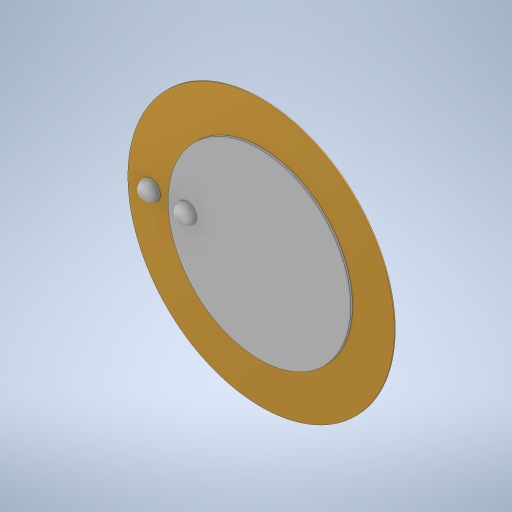
# Autodesk Inventor part: Piezo
Saved by Autodesk Inventor 2023 (Build 270158000, 158)
## iProperties
Created: 2023-02-27
Part Number: Piezo
Material: Generic
Document SubType Name: Modeling
Designer: maste
Density: 1 g/cm^3
Appearance: Default
Author: maste
Autodesk Inventor part; units mm, degrees
ref_plane "YZ Plane" through (0, 0, 0) normal (1, 0, 0) x (0, 1, 0)
ref_plane "XZ Plane" through (0, 0, 0) normal (0, 1, 0) x (-1, 0, 0)
ref_plane "XY Plane" through (0, 0, 0) normal (0, 0, 1) x (1, 0, 0)
sketch "Sketch1" plane through (0, 0, 0) normal (0, 0, 1) x (1, 0, 0)
  circle A0 centre (0, 0) radius 17.5
  dimension "d0" = 35
  constraints: 1 centre point, 1 coincident
  measures "d0" diameter of A0
extrude "Extrusion1" add sketch "Sketch1" along normal blind 0.13
sketch "Sketch2" plane through (0, 0, 0.13) normal (0, 0, 1) x (1, 0, 0)
  circle A0 centre (0, 0) radius 12
  dimension "d3" = 24
  constraints: 1 centre point, 1 coincident
  measures "d3" diameter of A0
extrude "Extrusion2" add sketch "Sketch2" along normal blind 0.22
sketch "Sketch3" plane through (0, 0, 0.13) normal (0, 0, 1) x (1, 0, 0)
  circle A0 centre (0, 0) radius 17.5 projected
  line L0 (-17.5, 0) -> (-14.5, 0)
  circle A1 centre (-14.5, 0) radius 1.25
  line L1 (-14.5, 0) -> (-13.25, 0)
  point P0 (-15.75, 0)
  dimension "d7" = 2.5
  dimension "d6" = 3
  constraints: 4 end point, 2 horizontal, 1 coincident, 1 horizontal alignment, 4 other
  measures "d6" distance of L0.start L0.end
revolve "Revolution1" add sketch "Sketch3" angle 180 about axis through (-17.5, 0, 0.13) along (1, 0, 0) picked at (-14.1156, 0.7325) contours A1 L1 L0
sketch "Sketch4" plane through (0, 0, 0.35) normal (0, 0, 1) x (1, 0, 0)
  circle A0 centre (-14.5, 0) radius 1.25 projected
  circle A1 centre (0, 0) radius 12 projected
  circle A2 centre (0, 0) radius 17.5 projected
  circle A3 centre (0, 0) radius 17.5 projected
  line L0 (-17.5, 0) -> (-9.5, 0)
  circle A4 centre (-9.5, 0) radius 1.25
  line L1 (-9.5, 0) -> (-8.25, 0)
  point P0 (-10.75, 0)
  dimension "d10" = 2.5
  dimension "d9" = 8
  constraints: 4 end point, 2 horizontal, 1 coincident, 1 horizontal alignment, 4 other
  measures "d9" distance of L0.start L0.end
revolve "Revolution2" add sketch "Sketch4" angle 180 about axis through (-17.5, 0, 0.35) along (1, 0, 0) picked at (-9.1156, 0.7325) contours A4 L1 L0
body "Solid1"
